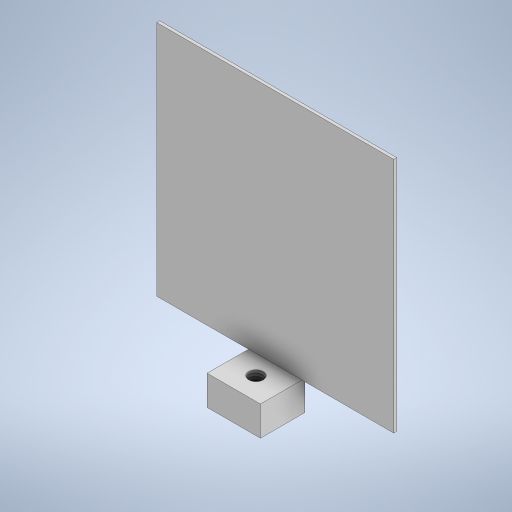
# Autodesk Inventor part: basicdifuser
Saved by Autodesk Inventor 2023 (Build 270158000, 158)
## iProperties
Created: 2022-05-18
Part Number: basicdifuser
Material: Generisch
Document SubType Name: Modeling
Designer: Tim Stechel
Density: 1 g/cm^3
Appearance: Vorgabe
Author: Tim Stechel
Autodesk Inventor part; units mm, degrees
ref_plane "YZ Plane" through (0, 0, 0) normal (1, 0, 0) x (0, 1, 0)
ref_plane "XZ Plane" through (0, 0, 0) normal (0, 1, 0) x (-1, 0, 0)
ref_plane "XY Plane" through (0, 0, 0) normal (0, 0, 1) x (1, 0, 0)
sketch "Skizze1" plane through (0, 0, 0) normal (0, 0, 1) x (1, 0, 0)
  line L0 (-20, 20) -> (20, 20)
  line L1 (20, 20) -> (20, -20)
  line L2 (20, -20) -> (-20, -20)
  line L3 (-20, -20) -> (-20, 20)
  line L4 (0, 20) -> (0, -20)
  line L5 (-20, 0) -> (20, 0)
  point P0 (0, 0)
  point P1 (0, 0)
  point P2 (-20, 0)
  point P3 (0, 0)
  point P4 (20, 0)
  dimension "d1" = 40
  dimension "d2" = 40
  constraints: 12 end point, 6 midpoint, 2 coincident, 2 parallel, 2 perpendicular, 1 horizontal, 2 other
  measures "d1" distance of L0.start L0.end
  measures "d2" distance of L0.end L1.end
extrude "Extrusion1" add sketch "Skizze1" along normal blind 0.5
sketch "Skizze2" plane through (0, 0, 0.5) normal (0, 0, 1) x (1, 0, 0)
  line L0 (-20, -20) -> (20, -20) projected
  line L1 (-4.5, -20) -> (4.5, -20)
  line L2 (4.5, -20) -> (4.5, -25)
  line L3 (4.5, -25) -> (-4.5, -25)
  line L4 (-4.5, -25) -> (-4.5, -20)
  line L5 (0, -20) -> (0, -25)
  point P0 (0, 0)
  dimension "d5" = 5
  dimension "d6" = 9
  constraints: 10 end point, 2 midpoint, 2 parallel, 2 perpendicular, 1 horizontal, 1 point on line, 1 other
  measures "d5" distance of L1.end L2.end
  measures "d6" distance of L2.end L3.end
extrude "Extrusion2" add sketch "Skizze2" along normal blind 7 and the other way blind 0.5
sketch "Skizze3" plane through (-4.5, -20, 0.5) normal (0, 1, 0) x (1, 0, 0)
  line L0 (0, -7) -> (0, 0) projected
  line L1 (9, 0.5) -> (0, 0.5) projected
  line L2 (0, -7) -> (9, 0.5)
  line L3 (9, 0.5) -> (9, -6.5)
  line L4 (9, -6.5) -> (0, 0)
  circle A0 centre (4.5, -3.25) radius 0.5388
  point P0 (4.5, 0.5)
  point P1 (0, 0.5)
  constraints: 6 end point, 1 centre point, 1 midpoint, 1 vertical, 1 other
hole "Bohrung1" at (0, -20, 3.75) direction (0, -1, 0) diameter 2.459 end through all thread size "M3x0.5" class "6H" standard "ISO Metric profile"
equation "\"d2\" = d1"
